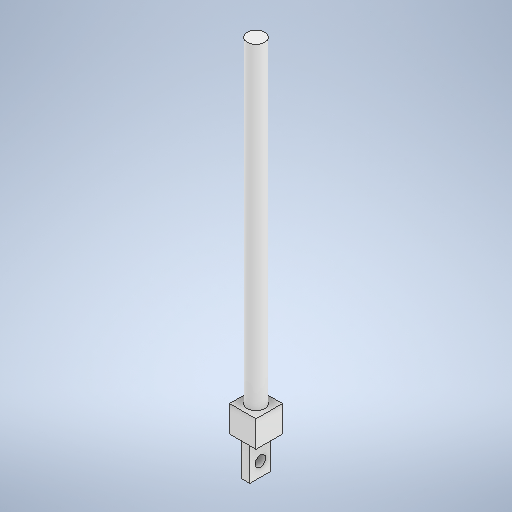
# Autodesk Inventor part: pendulum
Saved by Autodesk Inventor 2025.3 (Build 293356000, 356)
## iProperties
Created: 2025-07-22
Part Number: pendulum
Material: Plástico ABS
Document SubType Name: Modeling
Designer: KEVIN
Density: 1.06 g/cm^3
Appearance: Suave - Blanco
Mass: 70.8267 g
Surface Area: 154.565 cm^2
Volume: 66.8177 cm^3
Author: KEVIN
Autodesk Inventor part; units mm, degrees
ref_plane "YZ Plane" through (0, 0, 0) normal (1, 0, 0) x (0, 1, 0)
ref_plane "XZ Plane" through (0, 0, 0) normal (0, 1, 0) x (-1, 0, 0)
ref_plane "XY Plane" through (0, 0, 0) normal (0, 0, 1) x (1, 0, 0)
sketch "Boceto3" plane through (0, 0, 0) normal (0, 1, 0) x (-1, 0, 0)
  circle A0 centre (0, 0) radius 5
  dimension "d21" = 10
  constraints: 1 centre point, 1 coincident
  measures "d21" diameter of A0
extrude "Extrusión2" add sketch "Boceto3" along normal blind 180
sketch "Boceto4" plane through (0, 0, 0) normal (0, -1, 0) x (1, 0, 0)
  line L0 (-7.5, -7.5) -> (7.5, -7.5)
  line L1 (7.5, -7.5) -> (7.5, 7.5)
  line L2 (7.5, 7.5) -> (-7.5, 7.5)
  line L3 (-7.5, 7.5) -> (-7.5, -7.5)
  line L4 (-7.5, -7.5) -> (7.5, 7.5) construction
  line L5 (7.5, -7.5) -> (-7.5, 7.5) construction
  point P0 (0, 0)
  dimension "d24" = 15
  dimension "d25" = 15
  constraints: 12 end point, 2 midpoint, 2 parallel, 1 horizontal, 1 perpendicular
  measures "d24" distance of L2.end L1.end
  measures "d25" distance of L1.end L0.end
extrude "Extrusión3" add sketch "Boceto4" along normal blind 15
sketch "Boceto5" plane through (0, -15, 0) normal (0, -1, 0) x (1, 0, 0)
  line L0 (2.5, 6) -> (-2.5, 6)
  line L1 (-2.5, 6) -> (-2.5, -6)
  line L2 (-2.5, -6) -> (2.5, -6)
  line L3 (2.5, -6) -> (2.5, 6)
  line L4 (2.5, 6) -> (-2.5, -6) construction
  line L5 (-2.5, 6) -> (2.5, -6) construction
  point P0 (0, 0)
  dimension "d28" = 5
  dimension "d29" = 12
  constraints: 12 end point, 2 midpoint, 2 parallel, 1 horizontal, 1 perpendicular
  measures "d28" distance of L2.end L1.end
  measures "d29" distance of L1.end L0.end
extrude "Extrusión4" add sketch "Boceto5" along normal blind 20
sketch "Boceto6" plane through (2.5, -15, 6) normal (1, 0, 0) x (0, 0, -1)
  line L0 (12, -20) -> (0, -20) projected
  line L1 (6, -20) -> (6, -12)
  circle A0 centre (6, -12) radius 3
  point P0 (6, 15)
  dimension "d32" = 8
  dimension "d33" = 6
  constraints: 2 end point, 1 centre point, 1 coincident, 1 midpoint, 1 vertical
  measures "d32" distance of L1.start L1.end
  measures "d33" diameter of A0
extrude "Extrusión5" cut sketch "Boceto6" against normal blind 20
